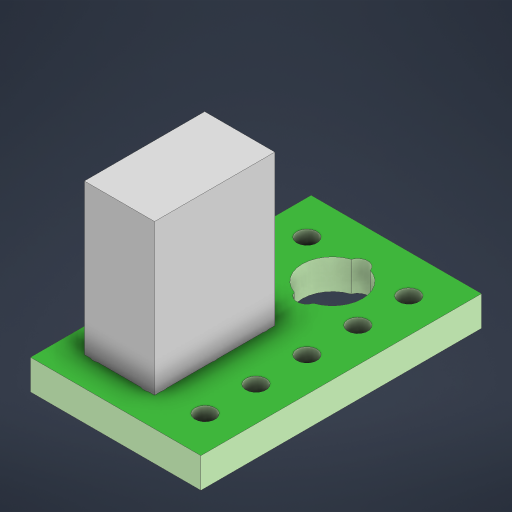
# Autodesk Inventor part: qre_module_V2
Saved by Autodesk Inventor 2024 (Build 280153000, 153)
## iProperties
Created: 2024-03-01
Part Number: qre_module_V2
Material: Všeobecné
Document SubType Name: Modeling
Designer: jaryj
Density: 1 g/cm^3
Appearance: Výchozí
Author: jaryj
Autodesk Inventor part; units mm, degrees
ref_plane "YZ Plane" through (0, 0, 0) normal (1, 0, 0) x (0, 1, 0)
ref_plane "XZ Plane" through (0, 0, 0) normal (0, 1, 0) x (-1, 0, 0)
ref_plane "XY Plane" through (0, 0, 0) normal (0, 0, 1) x (1, 0, 0)
sketch "Náčrt1" plane through (0, 0, 0) normal (0, 1, 0) x (-1, 0, 0)
  line L0 (4.25, 7) -> (-4.25, 7)
  line L1 (-4.25, 7) -> (-4.25, -7)
  line L2 (-4.25, -7) -> (4.25, -7)
  line L3 (4.25, -7) -> (4.25, 7)
  line L4 (4.25, 7) -> (-4.25, -7) construction
  line L5 (-4.25, 7) -> (4.25, -7) construction
  line L6 (2.54, 5.08) -> (-2.54, 5.08) construction
  line L7 (-2.54, 5.08) -> (-2.54, -5.08) construction
  line L8 (-2.54, -5.08) -> (2.54, -5.08) construction
  line L9 (2.54, -5.08) -> (2.54, 5.08) construction
  line L10 (2.54, 5.08) -> (-2.54, -5.08) construction
  line L11 (-2.54, 5.08) -> (2.54, -5.08) construction
  circle A0 centre (2.54, 5.08) radius 0.5
  circle A1 centre (2.54, 2.54) radius 0.5
  circle A2 centre (2.54, 0) radius 0.5
  circle A3 centre (2.54, -2.54) radius 0.5
  circle A4 centre (2.54, -5.08) radius 0.5
  circle A5 centre (0, 5.08) radius 0.5
  circle A6 centre (0, 2.54) radius 0.5
  circle A7 centre (0, 0) radius 0.5
  circle A8 centre (0, -2.54) radius 0.5
  circle A9 centre (0, -5.08) radius 0.5
  circle A10 centre (-2.54, 5.08) radius 0.5
  circle A11 centre (-2.54, 2.54) radius 0.5
  circle A12 centre (-2.54, 0) radius 0.5
  circle A13 centre (-2.54, -2.54) radius 0.5
  circle A14 centre (-2.54, -5.08) radius 0.5
  line L12 (0, -2.54) -> (0, -5.08) construction
  circle A15 centre (0, -3.81) radius 1.5
  point P0 (0, 0)
  point P1 (0.4762, -5.2324)
  point P2 (-0.4762, -5.2324)
  point P3 (-0.4762, -2.3876)
  point P4 (0.4762, -2.3876)
  dimension "d0" = 8.5
  dimension "d1" = 14
  dimension "d2" = 5.08
  dimension "d3" = 10.16
  dimension "d4" = 1
  dimension "d7" = 2.54
  dimension "d10" = 2.54
  dimension "d13" = 3
  constraints: 26 end point, 16 centre point, 5 midpoint, 4 parallel, 3 horizontal, 2 perpendicular, 2 vertical, 1 coincident, 28 other
  measures "d0" distance between parallel lines of L1 L3
  measures "d1" distance of L0.end L1.end
  measures "d2" distance of L6.start L6.end
  measures "d3" distance of L6.end L7.end
  measures "d4" diameter of A0
  measures "d7" distance of A0.centre A1.centre
  measures "d10" distance of A0.centre A5.centre
  measures "d13" diameter of A15
extrude "Vysunutí1" add sketch "Náčrt1" along normal blind 1.5
sketch "Náčrt2" plane through (0, 0, 0) normal (0, -1, 0) x (1, 0, 0)
  circle A0 centre (0, 2.54) radius 0.5 construction
  circle A1 centre (-2.54, 2.54) radius 0.5 construction
  line L0 (0, 2.54) -> (-2.54, 2.54) construction
  line L1 (0.48, 5.54) -> (-3.02, 5.54)
  line L2 (-3.02, 5.54) -> (-3.02, -0.46)
  line L3 (-3.02, -0.46) -> (0.48, -0.46)
  line L4 (0.48, -0.46) -> (0.48, 5.54)
  line L5 (0.48, 5.54) -> (-3.02, -0.46) construction
  line L6 (-3.02, 5.54) -> (0.48, -0.46) construction
  point P0 (0, 0)
  point P1 (-1.27, 2.54)
  dimension "d16" = 6
  dimension "d17" = 3.5
  constraints: 14 end point, 3 midpoint, 2 horizontal, 2 parallel, 1 perpendicular
  measures "d16" distance of L3.end L1.start
  measures "d17" distance of L1.start L1.end
extrude "Vysunutí2" add sketch "Náčrt2" against normal blind 9
